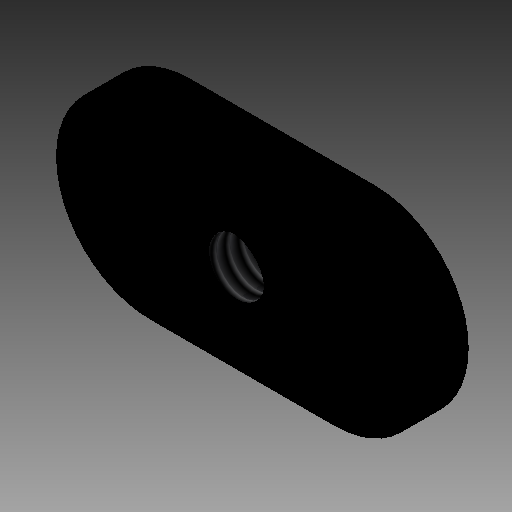
# Autodesk Inventor part: 3275
Saved by Autodesk Inventor 2019 (Build 230136000, 136)
## iProperties
Category: PARTsolutions
Company: 8020
Created: 2018-10-13
Part Number: 3275
Material: Generic
Catalog Web Link: www.cadenas.de
Description: 3275, 3276, 3675, 3382, 3785, 3859, 3686, 3286, 3786, 3836, 3676, 3278, 3778, 3838, 3678-Slide-In Economy T-Nuts
Vendor: 8020
Document SubType Name: Modeling
Designer: psadmin
Manufacturer: 8020
Mass: 0.518994 g
Surface Area: 6.05758 cm^2
Volume: 0.518994 cm^3
Density: 1 g/cm^3
Appearance: PSOLRGB-0-0-0
PSOL_IDENT_0: {$CADENAS_DATA\23d-libs\8020\inch\fastening_options\3275.prj},230 {VTYP=3D},{NB=3275},{LINA=3275},{N
PSOL_IDENT_1: N=3275, 3276, 3675, 3382, 3785, 3859, 3686, 3286, 3786, 3836, 3676, 3278, 3778, 3838, 3678},{DATE=02
PSOL_IDENT_2: .07.2018 05:48:01},{GEOMDATE=12.07.2017 13:43:48},{VERSION=},{LINEID=20},{WBVAR=},{WBNUMERIC=}  {NB=
PSOL_IDENT_3: 3275},{LINA=3275},{KT=DUMMY},{PN=3275},{NO=1},{NS=Style 1},{A=0.443},{B=0.875},{C=0.094},{D=8-32 Cen
PSOL_IDENT_4: tered},{M=0.1640},{FIN=Black Zinc},{W=.008},{COL=0.00,0.00,0.00,0.00},{X=0.203},{Y=0.030},{Z=0.0000}
PSOL_IDENT_5: ,{R=0.2215}
NN: 3275, 3276, 3675, 3382, 3785, 3859, 3686, 3286, 3786, 3836, 3676, 3278, 3778, 3838, 3678
NT: Slide-In Economy T-Nuts
NB: 3275
NBSYN: $PN.
LINA: 3275
PN: 3275
NS: Style 1
A: 0.443
B: 0.875
C: 0.094
D: 8-32 Centered
FIN: Black Zinc
W: .008
SUPPLIER: 8020
ARTICLENO: 3275
BOMINFO: 3275
CREATOR: CADENAS GmbH
d7: 0.000 in
d8: 0.000 in
Title: 3275
Author: Cadenas PARTsolutions
Comments: Slide-In Economy T-Nuts
Autodesk Inventor part; units mm, degrees
sketch "Sketch_1" plane through (0, 0, 0) normal (0, 0, 1) x (1, 0, 0)
  arc A0 (-5.4864, 5.6261) -> (-5.4864, -5.6261) centre (-5.4864, 0) ccw
  line L0 (-5.4864, -5.6261) -> (5.4864, -5.6261)
  arc A1 (5.4864, -5.6261) -> (5.4864, 5.6261) centre (5.4864, 0) ccw
  line L1 (5.4864, 5.6261) -> (-5.4864, 5.6261)
  constraints: 4 end point, 4 point on circle, 2 centre point
extrude "Extrusion1" add sketch "Sketch_1" along normal mid plane 2.3876
sketch "Sketch_3" plane through (0, 0, 0) normal (0, 0, 1) x (1, 0, 0)
  circle A0 centre (0, 0) radius 2.5781
  constraints: 1 centre point
extrude "Extrusion2" add sketch "Sketch_3" along normal blind 1.9558
sketch "Sketch_4" plane through (0, 0, 0) normal (1, 0, 0) x (0, 1, 0)
  line L0 (0, -1.1938) -> (0, 1.9558)
  line L1 (0, 1.9558) -> (2.0828, 1.9558)
  line L2 (2.0828, 1.9558) -> (1.6535, 1.5265)
  line L3 (1.6535, 1.5265) -> (1.6535, -0.7645)
  line L4 (1.6535, -0.7645) -> (2.0828, -1.1938)
  line L5 (2.0828, -1.1938) -> (0, -1.1938)
  line L6 (0, -1.1938) -> (0, 1.9558)
  constraints: 14 end point
revolve "Revolution1" cut sketch "Sketch_4" angle 360 about axis through (0, 0, -1.1938) along (0, 0, -1)
thread "Thread1" size "8-32 UNC" class "2B" standard "ANSI Unified Screw Threads" full length
ref_plane "tnut_XY" through (0, 0, -1.1938) normal (0, 0, 1) x (1, 0, 0)
ref_plane "tnut_YZ" through (0, 0, -1.1938) normal (1, 0, 0) x (0, 1, 0)
ref_plane "tnut_ZX" through (0, 0, -1.1938) normal (0, 1, 0) x (0, 0, 1)
ref_plane "tnut1_XY" through (0, 0, 1.1938) normal (0, 0, 1) x (1, 0, 0)
ref_plane "tnut1_YZ" through (0, 0, 1.1938) normal (1, 0, 0) x (0, 1, 0)
ref_plane "tnut1_ZX" through (0, 0, 1.1938) normal (0, 1, 0) x (0, 0, 1)
body "Solid1"
